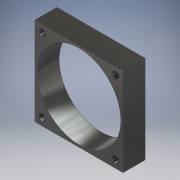
# Autodesk Inventor part: Fan
Saved by Autodesk Inventor 2017 (Build 210142000, 142)
## iProperties
Created: 2021-05-31
Part Number: Fan
Material: Silicon Nitride
Document SubType Name: Modeling
Designer: Win240
Mass: 46.8302 g
Surface Area: 91.1667 cm^2
Volume: 14.7265 cm^3
Density: 3.18 g/cm^3
Appearance: Chrome - Polished Black
Author: Win240
Autodesk Inventor part; units mm, degrees
ref_plane "YZ Plane" through (0, 0, 0) normal (1, 0, 0) x (0, 1, 0)
ref_plane "XZ Plane" through (0, 0, 0) normal (0, 1, 0) x (-1, 0, 0)
ref_plane "XY Plane" through (0, 0, 0) normal (0, 0, 1) x (1, 0, 0)
sketch "Sketch1" plane through (0, 0, 0) normal (0, 0, 1) x (1, 0, 0)
  line L0 (-30, -30) -> (30, -30)
  line L1 (30, -30) -> (30, 30)
  line L2 (30, 30) -> (-30, 30)
  line L3 (-30, 30) -> (-30, -30)
  line L4 (-30, -30) -> (30, 30) construction
  line L5 (30, -30) -> (-30, 30) construction
  line L6 (-25, 25) -> (25, 25) construction
  line L7 (25, 25) -> (25, -25) construction
  line L8 (25, -25) -> (-25, -25) construction
  line L9 (-25, -25) -> (-25, 25) construction
  circle A0 centre (-25, 25) radius 2.3
  circle A1 centre (25, 25) radius 2.3
  circle A2 centre (25, -25) radius 2.3
  circle A3 centre (-25, -25) radius 2.3
  circle A4 centre (0, 0) radius 28.5
  dimension "d0" = 50
  dimension "d1" = 60
  dimension "d2" = 4.6
  dimension "d3" = 57
  constraints: 20 end point, 5 centre point, 5 coincident, 4 parallel, 3 equal radius, 3 perpendicular, 3 point on line, 2 horizontal, 2 midpoint
  measures "d0" distance of L6.start L6.end
  measures "d1" distance of L1.end L2.end
  measures "d2" diameter of A0
  measures "d3" diameter of A4
extrude "Extrusion1" add sketch "Sketch1" along normal blind 15
body "Solid1"
